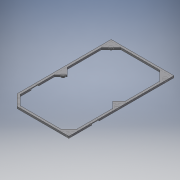
# Autodesk Inventor part: Backplate
Saved by Autodesk Inventor 2016 SP2 (Build 200236200, 236)
## iProperties
Created: 2018-06-10
Part Number: Backplate
Material: Generisch
Document SubType Name: Modeling
Designer: Nils
Density: 1 g/cm^3
Appearance: Vorgabe
Author: Nils
Autodesk Inventor part; units mm, degrees
ref_plane "YZ Plane" through (0, 0, 0) normal (1, 0, 0) x (0, 1, 0)
ref_plane "XZ Plane" through (0, 0, 0) normal (0, 1, 0) x (-1, 0, 0)
ref_plane "XY Plane" through (0, 0, 0) normal (0, 0, 1) x (1, 0, 0)
sketch "Skizze1" plane through (0, 0, 0) normal (0, 0, 1) x (1, 0, 0)
  line L0 (42.6168, 71.3457) -> (-42.6168, 71.3457) projected
  line L1 (-42.6168, 71.3457) -> (-42.6168, -71.3457) projected
  line L2 (42.6168, -71.3457) -> (42.6168, 71.3457) projected
  line L3 (-42.6168, -71.3457) -> (42.6168, -71.3457) projected
  line L4 (-18, -68.3457) -> (28.5457, -68.3457)
  line L5 (28.5457, -68.3457) -> (39.6168, -57.2746)
  line L6 (39.6168, -57.2746) -> (39.6168, -8.6569)
  line L7 (39.6168, 8.6569) -> (39.6168, 55.2746)
  line L8 (39.6168, 55.2746) -> (26.5457, 68.3457)
  line L9 (26.5457, 68.3457) -> (-26.5457, 68.3457)
  line L10 (-26.5457, 68.3457) -> (-39.6168, 55.2746)
  line L11 (-39.6168, 55.2746) -> (-39.6168, 8.6569)
  line L12 (-39.6168, 8.6569) -> (-30.9599, 0)
  line L13 (-30.9599, 0) -> (-39.6168, -8.6569)
  line L14 (-39.6168, -8.6569) -> (-39.6168, -55.103)
  line L15 (-39.6168, -55.103) -> (-26.3742, -68.3457)
  line L16 (-26.3742, -68.3457) -> (-18, -68.3457)
  line L17 (-42.6168, -56.3457) -> (-27.6168, -71.3457)
  circle A0 centre (37.6168, -66.3457) radius 2.5 construction
  circle A1 centre (36.6168, 0) radius 2.5 construction
  circle A2 centre (-36.6168, 0) radius 2.5 construction
  circle A3 centre (37.6168, -66.3457) radius 2.5 construction
  circle A4 centre (36.6168, 65.3457) radius 2.5 construction
  circle A5 centre (-36.6168, 65.3457) radius 2.5 construction
  line L18 (39.6168, -8.6569) -> (30.9599, 0)
  line L19 (30.9599, 0) -> (39.6168, 8.6569)
  point P0 (0, 0)
  dimension "d0" = 3
  dimension "d1" = 3
  dimension "d2" = 3
  dimension "d3" = 3
  dimension "d4" = 5
  dimension "d5" = 45
  dimension "d6" = 5
  dimension "d7" = 45
  dimension "d8" = 4
  dimension "d9" = 4
  dimension "d10" = 4
  dimension "d11" = 4
  dimension "d12" = 5
  dimension "d13" = 3
  dimension "d14" = 15
  constraints: 32 end point, 7 point on line, 6 parallel, 4 perpendicular, 1 collinear, 1 horizontal
  measures "d0" distance between parallel lines of L4 L3
  measures "d1" distance between parallel lines of L2 L6
  measures "d2" distance between parallel lines of L0 L9
  measures "d3" distance between parallel lines of L1 L11
  measures "d4" distance from line of A4.centre L8
  measures "d5" angle of L2 L8
  measures "d6" distance from line of A0.centre L5
  measures "d7" angle of L3 L5
  measures "d8" distance from line of L19 A1.centre
  measures "d9" distance from line of L18 A1.centre
  measures "d10" distance from line of L12 A2.centre
  measures "d11" distance from line of L13 A2.centre
  measures "d12" distance from line of L10 A5.centre
  measures "d13" distance between parallel lines of L17 L15
  measures "d14" distance of L17.end L1.end
extrude "Extrusion1" add sketch "Skizze1" along normal blind 2.5 contours L2 L3 L17 L1 L0
sketch "Skizze2" plane through (0, 0, 0) normal (0, 0, -1) x (-1, 0, 0)
  circle A0 centre (-36.6168, 65.3457) radius 2.4 projected
  circle A1 centre (36.6168, 65.3457) radius 2.4 projected
  circle A2 centre (36.6168, 0) radius 2.4 projected
  circle A3 centre (-36.6168, 0) radius 2.4 projected
  circle A4 centre (-37.6168, -66.3457) radius 2.4 projected
  point P0 (0, 0)
extrude "Extrusion2" add sketch "Skizze2" along normal blind 2.5
sketch "Skizze3" plane through (0, 0, 0) normal (0, 0, -1) x (-1, 0, 0)
  line L0 (42.6168, 71.3457) -> (42.6168, -56.3457) projected
  line L1 (39.6168, -8.6569) -> (39.6168, -55.103) projected
  line L2 (42.6168, -40.103) -> (39.6168, -40.103)
  line L3 (39.6168, -40.103) -> (39.6168, -30.103)
  line L4 (39.6168, -30.103) -> (42.6168, -30.103)
  line L5 (42.6168, -30.103) -> (42.6168, -40.103)
  line L6 (-39.6168, -57.2746) -> (-39.6168, -8.6569) projected
  line L7 (-42.6168, -71.3457) -> (-42.6168, 71.3457) projected
  line L8 (-39.6168, -40.103) -> (-42.6168, -40.103)
  line L9 (-42.6168, -40.103) -> (-42.6168, -30.103)
  line L10 (-42.6168, -30.103) -> (-39.6168, -30.103)
  line L11 (-39.6168, -30.103) -> (-39.6168, -40.103)
  line L12 (39.6168, -55.103) -> (26.3742, -68.3457) projected
  line L13 (29.7173, -65.0025) -> (36.7884, -57.9315)
  line L14 (26.3742, -68.3457) -> (39.6168, -55.103) projected
  line L15 (36.7884, -57.9315) -> (38.9097, -60.0528)
  line L16 (42.6168, -56.3457) -> (27.6168, -71.3457) projected
  line L17 (38.9097, -60.0528) -> (31.8386, -67.1239)
  line L18 (29.7173, -65.0025) -> (31.8386, -67.1239)
  point P0 (0, 0)
  dimension "d19" = 10
  dimension "d20" = 15
  dimension "d21" = 10
  dimension "d22" = 4
  constraints: 24 end point, 10 point on line, 4 parallel, 4 perpendicular, 2 horizontal
  measures "d19" distance between parallel lines of L15 L18
  measures "d20" distance from line of L1.end L2
  measures "d21" distance between parallel lines of L2 L4
  measures "d22" distance from line of L1.end L15
extrude "Extrusion3" cut sketch "Skizze3" against normal blind 1.5 contours L0 L2 L1 L4 | L16 L18 L12 L15 | L8 L7 L10 L6
equation "\"d1\" = d0"
equation "\"d2\" = d0"
equation "\"d3\" = d0"
